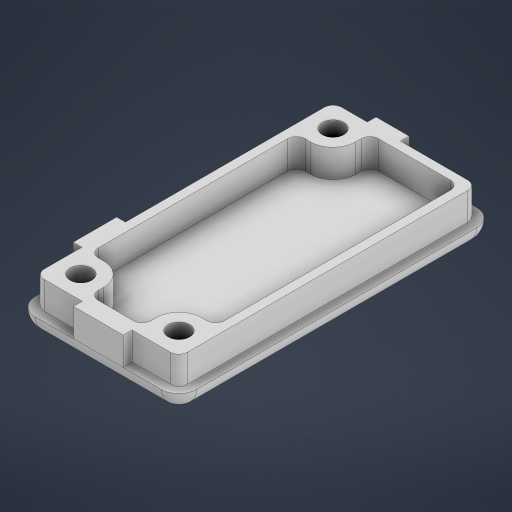
# Autodesk Inventor part: groundStation-Bottom
Saved by Autodesk Inventor 2024 (Build 280153000, 153)
## iProperties
Created: 2024-02-06
Part Number: groundStation-Bottom
Material: Generic
Document SubType Name: Modeling
Designer: madis
Density: 1 g/cm^3
Appearance: Default
Author: madis
Autodesk Inventor part; units mm, degrees
ref_plane "YZ Plane" through (0, 0, 0) normal (1, 0, 0) x (0, 1, 0)
ref_plane "XZ Plane" through (0, 0, 0) normal (0, 1, 0) x (-1, 0, 0)
ref_plane "XY Plane" through (0, 0, 0) normal (0, 0, 1) x (1, 0, 0)
sketch "Sketch1" plane through (0, 0, 0) normal (0, 1, 0) x (-1, 0, 0)
  line L0 (14.605, 25.4) -> (14.605, -25.4)
  line L1 (-14.605, 25.4) -> (-14.605, -25.4)
  line L2 (11.43, 28.575) -> (-11.43, 28.575)
  line L3 (11.43, -28.575) -> (-11.43, -28.575)
  arc A0 (14.605, 25.4) -> (11.43, 28.575) centre (11.43, 25.4) ccw
  arc A1 (-11.43, 28.575) -> (-14.605, 25.4) centre (-11.43, 25.4) ccw
  arc A2 (11.43, -28.575) -> (14.605, -25.4) centre (11.43, -25.4) ccw
  arc A3 (-14.605, -25.4) -> (-11.43, -28.575) centre (-11.43, -25.4) ccw
  point P0 (0, 0)
  dimension "d0" = 50.8
  dimension "d1" = 50.8
  dimension "d2" = 22.86
  dimension "d3" = 22.86
  dimension "d4" = 3.175
  dimension "d7" = 11.43
  dimension "d8" = 25.4
  dimension "d9" = 3.175
  constraints: 8 end point, 8 point on circle, 8 tangent, 4 centre point, 2 horizontal, 2 vertical, 1 other
  measures "d0" distance of L0.start L0.end
  measures "d1" distance of L1.start L1.end
  measures "d2" distance of L2.start L2.end
  measures "d3" distance of L3.start L3.end
  measures "d4" radius of A0
  measures "d7" horizontal distance of A2.centre point (0, 0)
  measures "d8" vertical distance of point (0, 0) A2.centre
  measures "d9" radius of A2
extrude "Extrusion1" add sketch "Sketch1" along normal blind 3.175
sketch "Sketch2" plane through (0, 3.175, 0) normal (0, 1, 0) x (1, 0, 0)
  line L0 (-13.0175, 25.4) -> (-13.0175, -25.4)
  line L1 (13.0175, 25.4) -> (13.0175, -25.4)
  line L2 (-11.43, 26.9875) -> (11.43, 26.9875)
  line L3 (-11.43, -26.9875) -> (11.43, -26.9875)
  arc A0 (-11.43, 26.9875) -> (-13.0175, 25.4) centre (-11.43, 25.4) ccw
  arc A1 (13.0175, 25.4) -> (11.43, 26.9875) centre (11.43, 25.4) ccw
  arc A2 (11.43, -26.9875) -> (13.0175, -25.4) centre (11.43, -25.4) ccw
  arc A3 (-13.0175, -25.4) -> (-11.43, -26.9875) centre (-11.43, -25.4) ccw
  circle A4 centre (-8.89, 22.86) radius 1.9431
  circle A5 centre (-8.89, -22.86) radius 1.9431
  circle A6 centre (8.89, -22.86) radius 1.9431
  arc A7 (-8.89, 18.7325) -> (-4.7625, 22.86) centre (-8.89, 22.86) ccw
  arc A8 (-4.7625, -22.86) -> (-8.89, -18.7325) centre (-8.89, -22.86) ccw
  arc A9 (-9.8425, 18.7325) -> (-11.43, 17.145) centre (-9.8425, 17.145) ccw
  line L4 (-9.8425, 18.7325) -> (-8.89, 18.7325)
  line L5 (-4.7625, 22.86) -> (-4.7625, 23.8125)
  arc A10 (-3.175, 25.4) -> (-4.7625, 23.8125) centre (-3.175, 23.8125) ccw
  arc A11 (11.43, 23.8125) -> (9.8425, 25.4) centre (9.8425, 23.8125) ccw
  line L6 (9.8425, 25.4) -> (-3.175, 25.4)
  arc A12 (9.8425, -18.7325) -> (11.43, -17.145) centre (9.8425, -17.145) ccw
  line L7 (11.43, -17.145) -> (11.43, 23.8125)
  line L8 (8.89, -18.7325) -> (9.8425, -18.7325)
  line L9 (-4.7625, -22.86) -> (-4.7625, -23.8125)
  arc A13 (-4.7625, -23.8125) -> (-3.175, -25.4) centre (-3.175, -23.8125) ccw
  line L10 (-3.175, -25.4) -> (3.175, -25.4)
  arc A14 (3.175, -25.4) -> (4.7427, -23.5628) centre (3.175, -23.8125) ccw
  line L11 (4.7625, -22.86) -> (4.7625, -23.8125)
  arc A15 (8.89, -18.7325) -> (4.7625, -22.86) centre (8.89, -22.86) ccw
  line L12 (-8.89, -18.7325) -> (-9.8425, -18.7325)
  arc A16 (-11.43, -17.145) -> (-9.8425, -18.7325) centre (-9.8425, -17.145) ccw
  line L13 (-11.43, 17.145) -> (-11.43, -17.145)
  line L14 (-14.605, 25.4) -> (-14.605, -25.4) projected
  line L15 (11.43, 28.575) -> (-11.43, 28.575) projected
  line L16 (14.605, -25.4) -> (14.605, 25.4) projected
  line L17 (-11.43, -28.575) -> (11.43, -28.575) projected
  line L18 (-4.5085, -26.9875) -> (4.5085, -26.9875)
  line L19 (4.5085, -26.9875) -> (4.5085, -28.575)
  line L20 (4.5085, -28.575) -> (-4.5085, -28.575)
  line L21 (-4.5085, -28.575) -> (-4.5085, -26.9875)
  line L22 (-14.605, -10.655) -> (-13.0175, -10.655)
  line L23 (-13.0175, -10.655) -> (-13.0175, -18.555)
  line L24 (-13.0175, -18.555) -> (-14.605, -18.555)
  line L25 (-14.605, -18.555) -> (-14.605, -10.655)
  line L26 (-6.81, 28.575) -> (-0.81, 28.575)
  line L27 (-0.81, 28.575) -> (-0.81, 26.9875)
  line L28 (-0.81, 26.9875) -> (-6.81, 26.9875)
  line L29 (-6.81, 26.9875) -> (-6.81, 28.575)
  point P0 (0, 0)
  point P1 (-4.5085, -28.575)
  dimension "d15" = 2.54
  dimension "d18" = 2.54
  dimension "d19" = 2.54
  dimension "d20" = 2.54
  dimension "d21" = 2.54
  dimension "d22" = 3.8862
  dimension "d24" = 3.8862
  dimension "d25" = 3.8862
  dimension "d40" = 1.5875
  dimension "d41" = 1.5875
  dimension "d43" = 2.54
  dimension "d44" = 1.5875
  dimension "d47" = 1.5875
  dimension "d50" = 1.5875
  dimension "d52" = 1.5875
  dimension "d53" = 1.5875
  dimension "d54" = 1.5875
  dimension "d56" = 1.5875
  dimension "d57" = 1.5875
  dimension "d58" = 1.5875
  dimension "d59" = 1.5875
  dimension "d60" = 1.5875
  dimension "d61" = 1.5875
  dimension "d62" = 1.5875
  dimension "d63" = 0
  dimension "d64" = 1.5875
  dimension "d65" = 1.5875
  dimension "d66" = 1.5875
  dimension "d67" = 1.5875
  dimension "d68" = 9.017
  dimension "d69" = 4.3815
  dimension "d70" = 4.305
  dimension "d71" = 7.9
  dimension "d72" = 2.08
  dimension "d73" = 6
  constraints: 52 end point, 30 tangent, 29 point on circle, 17 centre point, 10 horizontal, 7 coincident, 7 vertical, 6 parallel, 6 point on line, 3 perpendicular
  measures "d15" horizontal distance of point (-11.43, 25.4) A4.centre
  measures "d18" horizontal distance of point (-11.43, -25.4) A5.centre
  measures "d19" horizontal distance of point (-11.43, -25.4) A5.centre
  measures "d20" horizontal distance of point (11.43, -25.4) A6.centre
  measures "d21" horizontal distance of point (11.43, -25.4) A6.centre
  measures "d22" diameter of A4
  measures "d24" diameter of A5
  measures "d25" diameter of A6
  measures "d40" radius of A3
  measures "d41" radius of A2
  measures "d43" horizontal distance of point (-11.43, 25.4) A4.centre
  measures "d44" radius of A1
  measures "d47" radius of A0
  measures "d50" radius of A9
  measures "d52" radius of A10
  measures "d53" radius of A11
  measures "d54" distance between parallel lines of L2 L6
  measures "d56" radius of A12
  measures "d57" distance between parallel lines of L1 L7
  measures "d58" radius of A13
  measures "d59" radius of A14
  measures "d60" radius of A16
  measures "d61" distance between parallel lines of L0 L13
  measures "d62" distance between parallel lines of L3 L10
  measures "d63" vertical distance of A16.centre A12.centre
  measures "d64" distance between parallel lines of L14 L0
  measures "d65" distance between parallel lines of L15 L2
  measures "d66" distance between parallel lines of L16 L1
  measures "d67" distance between parallel lines of L17 L3
  measures "d68" distance between parallel lines of L19 L21
  measures "d69" distance from line of A5.centre L21
  measures "d70" distance from line of A5.centre L24
  measures "d71" distance between parallel lines of L24 L22
  measures "d72" distance from line of A4.centre L29
  measures "d73" distance between parallel lines of L27 L29
extrude "Extrusion2" add sketch "Sketch2" along normal blind 5.08
fillet "Fillet1" radius 3.175 8 edges at (13.6751, 0, 27.6451) (14.605, 0, 0) (13.6751, 0, -27.6451) (0, 0, -28.575) (-13.6751, 0, -27.6451) (-14.605, 0, 0) (-13.6751, 0, 27.6451) (0, 0, 28.575)
body "Solid1"
